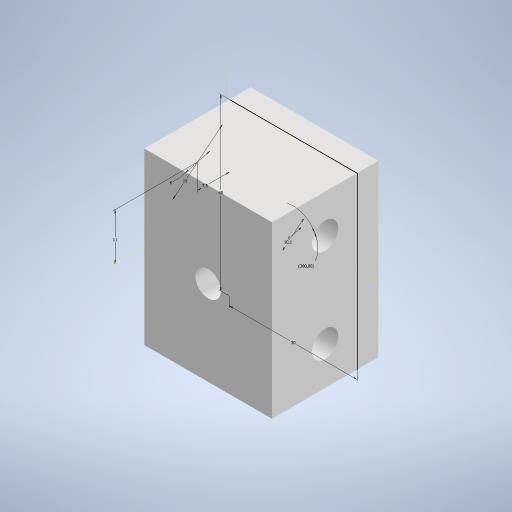
# Autodesk Inventor part: uMule-Uchwyt_koła
Saved by Autodesk Inventor 2024.2 (Build 282272000, 272)
## iProperties
Created: 2024-10-21
Part Number: uMule-Uchwyt_koła
Material: Ogólny
Document SubType Name: Modeling
Designer: owozn
Density: 1 g/cm^3
Appearance: Domyślna
Author: owozn
Autodesk Inventor part; units mm, degrees
ref_plane "YZ Plane" through (0, 0, 0) normal (1, 0, 0) x (0, 1, 0)
ref_plane "XZ Plane" through (0, 0, 0) normal (0, 1, 0) x (-1, 0, 0)
ref_plane "XY Plane" through (0, 0, 0) normal (0, 0, 1) x (1, 0, 0)
sketch "Szkic1" plane through (0, 0, 0) normal (0, 0, 1) x (1, 0, 0)
  line L0 (-21, 0) -> (21, 0) construction
  line L1 (0, -28) -> (0, 28) construction
  circle A0 centre (0, 0) radius 3
  circle A1 centre (0, 0) radius 5.05
  line L2 (15, 20) -> (-15, 20)
  line L3 (-15, 20) -> (-15, -20)
  line L4 (-15, -20) -> (15, -20)
  line L5 (15, -20) -> (15, 20)
  line L6 (15, 20) -> (-15, -20) construction
  line L7 (-15, 20) -> (15, -20) construction
  line L8 (5.05, 2.9156) -> (5.05, -2.9156)
  line L9 (0, 5.8312) -> (5.05, 2.9156)
  line L10 (-5.05, 2.9156) -> (0, 5.8312)
  line L11 (-5.05, -2.9156) -> (-5.05, 2.9156)
  line L12 (0, -5.8312) -> (-5.05, -2.9156)
  line L13 (5.05, -2.9156) -> (0, -5.8312)
  point P0 (5.05, -2.9156)
  dimension "d0" = 6
  dimension "d1" = 10.1
  dimension "d2" = 30
  dimension "d3" = 40
  dimension "d8" = 360
  constraints: 24 end point, 3 coincident, 2 centre point, 2 midpoint, 2 parallel, 1 horizontal, 1 perpendicular, 1 point on line, 1 tangent, 19 other
  measures "d0" diameter of A0
  measures "d1" diameter of A1
  measures "d2" distance of L4.end L3.end
  measures "d3" distance of L3.end L2.end
extrude "Wyciągnięcie proste1" add sketch "Szkic1" along normal blind 20 contours A1 | L8 L13 A1 | A1 L9 L8 | A1 L10 L9 | L13 L12 A1 | A1 L11 L10 | L12 L11 A1 | L5 L4 L3 L2
extrude "Wyciągnięcie proste2" add sketch "Szkic1" against normal blind 5 contours L5 L4 L3 L2
fillet "Zaokrąglenie1" radius 1 6 edges at (5.05, 0, -5) (2.525, 4.3734, -5) (-2.525, 4.3734, -5) (-5.05, 0, -5) (-2.525, -4.3734, -5) (2.525, -4.3734, -5)
sketch "Szkic2" plane through (-15, -20, 20) normal (-1, 0, 0) x (0, 0, 1)
  line L0 (-25, 0) -> (-25, 40) projected
  line L1 (-20, -8) -> (-20, 48) construction
  line L2 (-30.5, 20) -> (8, 20) construction
  circle A0 centre (-12.5, 31) radius 3
  circle A1 centre (-12.5, 9) radius 3
  circle A2 centre (-12.5, 31) radius 7.5
  circle A3 centre (-12.5, 9) radius 7.5
  point P0 (-20, 20)
  dimension "d14" = 6
  dimension "d15" = 7.5
  dimension "d16" = 11
  dimension "d17" = 15
  constraints: 4 centre point, 2 symmetric about line, 1 coincident, 2 other
  measures "d14" diameter of A0
  measures "d15" distance from line of L1 A0.centre
  measures "d16" distance from line of L2 A0.centre
  measures "d17" diameter of A2
extrude "Wyciągnięcie proste3" cut sketch "Szkic2" against normal through all contours A0 | A1
hole "Otwór1" at (-15, -11, 7.5) at (-15, 11, 7.5) direction (1, 0, 0) diameter 6.2 end through all
